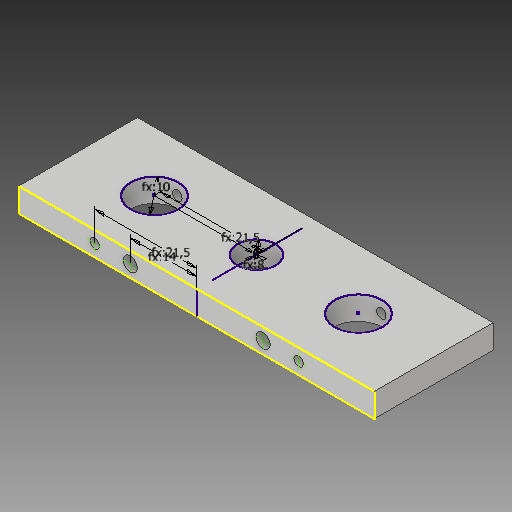
# Autodesk Inventor part: Placa2
Saved by Autodesk Inventor 2017 (Build 210142000, 142)
## iProperties
Part Number: Placa2
Material: Genérico
Document SubType Name: Modeling
Designer: osvaldo
Density: 1 g/cm^3
Appearance: Valor por defecto
Author: osvaldo
Autodesk Inventor part; units mm, degrees
ref_plane "YZ Plane" through (0, 0, 0) normal (1, 0, 0) x (0, 1, 0)
ref_plane "XZ Plane" through (0, 0, 0) normal (0, 1, 0) x (-1, 0, 0)
ref_plane "XY Plane" through (0, 0, 0) normal (0, 0, 1) x (1, 0, 0)
sketch "Boceto1" plane through (0, 0, 0) normal (0, 1, 0) x (-1, 0, 0)
  line L0 (-37.5, 12.5) -> (37.5, 12.5)
  line L1 (37.5, 12.5) -> (37.5, -12.5)
  line L2 (37.5, -12.5) -> (-37.5, -12.5)
  line L3 (-37.5, -12.5) -> (-37.5, 12.5)
  line L4 (-37.5, 12.5) -> (37.5, -12.5) construction
  line L5 (37.5, 12.5) -> (-37.5, -12.5) construction
  point P0 (0, 0)
  dimension "d4" = 25
  dimension "d5" = 75
  constraints: 12 end point, 2 midpoint, 2 parallel, 1 horizontal, 1 perpendicular
  measures "d4" distance of L0.end L1.end
  measures "d5" distance of L1.end L2.end
extrude "Extrusión1" add sketch "Boceto1" along normal blind 5
sketch "Boceto2" plane through (-37.5, 0, 12.5) normal (0, 0, 1) x (1, 0, 0)
  line L0 (75, 0) -> (0, 0) projected
  line L1 (75, 0) -> (75, 5) projected
  line L2 (0, 5) -> (75, 5) projected
  line L3 (0, 0) -> (0, 5) projected
  line L4 (37.5, 0) -> (37.5, 5)
  point P0 (23.5, 2.5)
  point P1 (16, 2.5)
  point P2 (51.5, 2.5)
  point P3 (59, 2.5)
  dimension "d12" = 14
  dimension "d13" = 21.5
  constraints: 2 end point, 2 symmetric about line, 1 midpoint
  measures "d12" distance from line of L4 point (23.5, 2.5)
  measures "d13" distance from line of L4 point (16, 2.5)
hole "Agujero1" at (-14, 2.5, 12.5) at (14, 2.5, 12.5) direction (0, 0, -1) diameter 3 end through all
hole "Agujero2" at (-21.5, 2.5, 12.5) at (21.5, 2.5, 12.5) direction (0, 0, -1) diameter 2 depth 20 tip angle 118
sketch "Boceto3" plane through (0, 5, 0) normal (0, 1, 0) x (1, 0, 0)
  circle A0 centre (-21.5, 0) radius 5
  line L0 (0, -9.1996) -> (0, 9.6209)
  circle A1 centre (21.5, 0) radius 5
  circle A2 centre (0, 0) radius 4
  dimension "d28" = 21.5
  dimension "d29" = 0
  dimension "d30" = 10
  dimension "d31" = 0
  dimension "d34" = 8
  dimension "d35" = 0
  dimension "d36" = 0
  constraints: 3 centre point, 2 end point, 1 symmetric about line, 1 vertical, 1 other
  measures "d28" distance of point (0, 0) A0.centre
  measures "d29" vertical distance of point (0, 0) A0.centre
  measures "d30" diameter of A0
  measures "d31" distance from line of L0 point (0, 0)
  measures "d34" diameter of A2
  measures "d35" distance of point (0, 0) A2.centre
  measures "d36" distance of point (0, 0) A2.centre
extrude "Extrusión2" cut sketch "Boceto3" against normal through all
equation "\"d4\" = 25 * scale"
equation "\"d5\" = 75 * scale"
equation "\"d2\" = 5 * scale"
equation "\"d12\" = 14 * scale"
equation "\"d13\" = 21.5 * scale"
equation "\"d28\" = 21.5 * scale"
equation "\"d30\" = 10 * scale"
equation "\"d34\" = 8 * scale"
equation "\"scale\" = 1"
